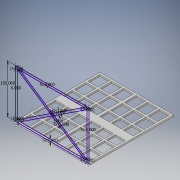
# Autodesk Inventor part: 4 Tape Measures Holder V2
Saved by Autodesk Inventor 2019 (Build 230136000, 136)
## iProperties
Created: 2018-12-28
Part Number: 4 Tape Measures Holder V2
Material: Generic
Document SubType Name: Modeling
Designer: ashle
Density: 1 g/cm^3
Appearance: Default
Author: ashle
Autodesk Inventor part; units mm, degrees
ref_plane "YZ Plane" through (0, 0, 0) normal (1, 0, 0) x (0, 1, 0)
ref_plane "XZ Plane" through (0, 0, 0) normal (0, 1, 0) x (-1, 0, 0)
ref_plane "XY Plane" through (0, 0, 0) normal (0, 0, 1) x (1, 0, 0)
sketch "Sketch1" plane through (0, 0, 0) normal (0, 1, 0) x (-1, 0, 0)
  line L0 (2743.2, 3327.4) -> (-2743.2, 3327.4)
  line L1 (-2743.2, 3327.4) -> (-2743.2, 3175)
  line L2 (-2743.2, 3175) -> (2743.2, 3175)
  line L3 (2743.2, 3175) -> (2743.2, 3327.4)
  line L4 (0, 5131.2687) -> (0, -6149.1862) construction
  line L5 (2743.2, 4620.3571) -> (2743.2, -4424.6448) construction
  line L6 (-2743.2, 4620.3571) -> (-2743.2, -5005.5165) construction
  line L7 (-3643.9458, -3175) -> (3603.587, -3175) construction
  line L8 (3452.6337, 3175) -> (-4564.2023, 3175) construction
  line L9 (-2743.2, 2243.6667) -> (-2743.2, 2091.2667)
  line L10 (2743.2, 2243.6667) -> (-2743.2, 2243.6667)
  line L11 (-2743.2, 2091.2667) -> (2743.2, 2091.2667)
  line L12 (2743.2, 2091.2667) -> (2743.2, 2243.6667)
  line L13 (-2743.2, 1159.9333) -> (-2743.2, 1007.5333)
  line L14 (2743.2, 1159.9333) -> (-2743.2, 1159.9333)
  line L15 (-2743.2, 1007.5333) -> (2743.2, 1007.5333)
  line L16 (2743.2, 1007.5333) -> (2743.2, 1159.9333)
  line L17 (-2743.2, -317.5) -> (2743.2, -317.5)
  line L18 (2743.2, -317.5) -> (2743.2, 317.5)
  line L19 (2743.2, 317.5) -> (-2743.2, 317.5)
  line L20 (-2743.2, 317.5) -> (-2743.2, -317.5)
  line L21 (-2743.2, -317.5) -> (2743.2, 317.5) construction
  line L22 (2743.2, -317.5) -> (-2743.2, 317.5) construction
  line L23 (-101.6, -3327.4) -> (101.6, -3327.4)
  line L24 (101.6, -3327.4) -> (101.6, 3327.4)
  line L25 (101.6, 3327.4) -> (-101.6, 3327.4)
  line L26 (-101.6, 3327.4) -> (-101.6, -3327.4)
  line L27 (-101.6, -3327.4) -> (101.6, 3327.4) construction
  line L28 (101.6, -3327.4) -> (-101.6, 3327.4) construction
  line L29 (3750.9383, 0) -> (-5642.9813, 0) construction
  line L30 (2743.2, -3327.4) -> (-2743.2, -3327.4)
  line L31 (-2743.2, -3327.4) -> (-2743.2, -3175)
  line L32 (-2743.2, -3175) -> (2743.2, -3175)
  line L33 (2743.2, -3175) -> (2743.2, -3327.4)
  line L34 (-2743.2, -2243.6667) -> (-2743.2, -2091.2667)
  line L35 (2743.2, -2243.6667) -> (-2743.2, -2243.6667)
  line L36 (-2743.2, -2091.2667) -> (2743.2, -2091.2667)
  line L37 (2743.2, -2091.2667) -> (2743.2, -2243.6667)
  line L38 (-2743.2, -1159.9333) -> (-2743.2, -1007.5333)
  line L39 (2743.2, -1159.9333) -> (-2743.2, -1159.9333)
  line L40 (-2743.2, -1007.5333) -> (2743.2, -1007.5333)
  line L41 (2743.2, -1007.5333) -> (2743.2, -1159.9333)
  line L42 (2895.6, 3327.4) -> (2743.2, 3327.4)
  line L43 (2743.2, 3327.4) -> (2743.2, -3327.4)
  line L44 (2743.2, -3327.4) -> (2895.6, -3327.4)
  line L45 (2895.6, -3327.4) -> (2895.6, 3327.4)
  line L46 (1803.4, 3327.4) -> (1803.4, -3327.4)
  line L47 (1955.8, -3327.4) -> (1955.8, 3327.4)
  line L48 (1955.8, 3327.4) -> (1803.4, 3327.4)
  line L49 (1803.4, -3327.4) -> (1955.8, -3327.4)
  line L50 (863.6, 3327.4) -> (863.6, -3327.4)
  line L51 (1016, -3327.4) -> (1016, 3327.4)
  line L52 (1016, 3327.4) -> (863.6, 3327.4)
  line L53 (863.6, -3327.4) -> (1016, -3327.4)
  line L54 (-2895.6, 3327.4) -> (-2743.2, 3327.4)
  line L55 (-2743.2, 3327.4) -> (-2743.2, -3327.4)
  line L56 (-2743.2, -3327.4) -> (-2895.6, -3327.4)
  line L57 (-2895.6, -3327.4) -> (-2895.6, 3327.4)
  line L58 (-1803.4, 3327.4) -> (-1803.4, -3327.4)
  line L59 (-1955.8, -3327.4) -> (-1955.8, 3327.4)
  line L60 (-1955.8, 3327.4) -> (-1803.4, 3327.4)
  line L61 (-1803.4, -3327.4) -> (-1955.8, -3327.4)
  line L62 (-863.6, 3327.4) -> (-863.6, -3327.4)
  line L63 (-1016, -3327.4) -> (-1016, 3327.4)
  line L64 (-1016, 3327.4) -> (-863.6, 3327.4)
  line L65 (-863.6, -3327.4) -> (-1016, -3327.4)
  point P0 (0, 0)
  point P1 (-1803.4, 3327.4)
  dimension "d0" = 5486.4
  dimension "d1" = 152.4
  dimension "d5" = 2743.2
  dimension "d6" = 3175
  dimension "d7" = 6350
  dimension "d10" = 1083.7333
  dimension "d15" = 635
  dimension "d16" = 203.2
  dimension "d19" = 2015.0667
  dimension "d20" = 2015.0667
  dimension "d21" = 152.4
  dimension "d24" = 939.8
  dimension "d29" = 1727.2
  dimension "d30" = 1727.2
  dimension "d32" = 939.8
  dimension "d33" = 1083.7333
  dimension "d36" = 152.4
  dimension "d37" = 152.4
  constraints: 132 end point, 28 symmetric about line, 8 collinear, 8 horizontal, 8 parallel, 4 midpoint, 4 perpendicular, 4 vertical, 36 other
  measures "d0" distance of L0.start L0.end
  measures "d1" distance of L2.end L0.start
  measures "d5" distance from line of point (0, 0) L1
  measures "d6" distance from line of point (0, 0) L2
  measures "d7" distance between parallel lines of L7 L8
  measures "d10" distance of L0.end L9.start
  measures "d15" distance between parallel lines of L17 L19
  measures "d16" distance between parallel lines of L26 L24
  measures "d19" distance between parallel lines of L14 L2
  measures "d20" distance between parallel lines of L40 L15
  measures "d21" distance of L42.start L42.end
  measures "d24" distance of L42.end L46.start
  measures "d29" distance between parallel lines of L43 L51
  measures "d30" distance between parallel lines of L62 L50
  measures "d32" distance between parallel lines of L58 L62
  measures "d33" distance between parallel lines of L40 L36
  measures "d36" distance between parallel lines of L35 L36
  measures "d37" distance between parallel lines of L59 L58
extrude "Extrusion1" add sketch "Sketch1" along normal blind 127 contours L3 L2 L47 L0 | L42 L45 L44 L33 L43 L37 L41 L18 L16 L12 L3 | L47 L2 L46 L0 | L46 L2 L51 L0 | L47 L10 L46 L2 | L12 L11 L47 L10 | L51 L2 L50 L0 | L47 L11 L46 L10 | L30 L47 L32 L33 | L50 L2 L24 L0 | L51 L10 L50 L2 | L46 L11 L51 L10 | L47 L14 L46 L11 | L16 L15 L47 L14 | L30 L46 L32 L47 | L24 L2 L26 L0 | L51 L11 L50 L10 | L47 L15 L46 L14 | L30 L51 L32 L46 | L32 L46 L35 L47 | L35 L47 L36 L37 | L26 L2 L62 L0 | L24 L10 L26 L2 | L50 L11 L24 L10 | L51 L14 L50 L11 | L46 L15 L51 L14 | L47 L19 L46 L15 | L18 L17 L47 L19 | L30 L50 L32 L51 | L35 L46 L36 L47 | L62 L2 L63 L0 | L24 L11 L26 L10 | L51 L15 L50 L14 | L47 L17 L46 L19 | L30 L24 L32 L50 | L32 L50 L35 L51 | L35 L51 L36 L46 | L36 L46 L39 L47 | L39 L47 L40 L41 | L63 L2 L58 L0 | L62 L10 L63 L2 | L26 L11 L62 L10 | L24 L14 L26 L11 | L50 L15 L24 L14 | L51 L19 L50 L15 | L46 L17 L51 L19 | L47 L40 L46 L17 | L23 L26 L32 L24 | L35 L50 L36 L51 | L39 L46 L40 L47 | L58 L2 L59 L0 | L62 L11 L63 L10 | L24 L15 L26 L14 | L51 L17 L50 L19 | L30 L62 L32 L26 | L32 L26 L35 L24 | L35 L24 L36 L50 | L36 L50 L39 L51 | L39 L51 L40 L46 | L59 L2 L1 L0 | L58 L10 L59 L2 | L63 L11 L58 L10 | L62 L14 L63 L11 | L26 L15 L62 L14 | L24 L19 L26 L15 | L50 L17 L24 L19 | L51 L40 L50 L17 | L30 L63 L32 L62 | L35 L26 L36 L24 | L39 L50 L40 L51 | L1 L55 L9 L13 L20 L38 L34 L31 L56 L57 L54 | L58 L11 L59 L10 | L62 L15 L63 L14 | L24 L17 L26 L19 | L35 L62 L36 L26 | L32 L63 L35 L62 | L30 L58 L32 L63 | L36 L26 L39 L24 | L39 L24 L40 L50 | L59 L11 L9 L10 | L58 L14 L59 L11 | L63 L15 L58 L14 | L62 L19 L63 L15 | L26 L17 L62 L19 | L24 L40 L26 L17 | L35 L63 L36 L62 | L30 L59 L32 L58 | L39 L26 L40 L24 | L58 L15 L59 L14 | L62 L17 L63 L19 | L39 L62 L40 L26 | L36 L63 L39 L62 | L35 L58 L36 L63 | L32 L59 L35 L58 | L30 L31 L32 L59 | L59 L15 L13 L14 | L58 L19 L59 L15 | L63 L17 L58 L19 | L62 L40 L63 L17 | L39 L63 L40 L62 | L35 L59 L36 L58 | L58 L17 L59 L19 | L39 L58 L40 L63 | L36 L59 L39 L58 | L35 L34 L36 L59 | L59 L17 L20 L19 | L58 L40 L59 L17 | L39 L59 L40 L58 | L39 L38 L40 L59
sketch "Sketch8" plane through (-2895.6, 0, 3327.4) normal (0, 0, 1) x (1, 0, 0)
  line L0 (5791.2, 127) -> (0, 127) construction
  line L1 (0, 127) -> (0, 3937)
  line L2 (0, 3937) -> (5791.2, 3937)
  line L3 (5791.2, 3937) -> (5791.2, 127)
  line L4 (5791.2, 127) -> (0, 3937) construction
  line L5 (0, 127) -> (5791.2, 3937) construction
  line L6 (0, 0) -> (0, 127) construction
  line L7 (5791.2, 0) -> (5791.2, 127) construction
  line L8 (5791.2, 127) -> (0, 127) construction
  line L9 (0, 127) -> (193.04, 127) construction
  line L10 (193.04, 127) -> (193.04, 254) construction
  line L11 (193.04, 254) -> (0, 254) construction
  line L12 (0, 254) -> (0, 127) construction
  line L13 (5791.2, 3937) -> (5598.16, 3937) construction
  line L14 (5598.16, 3937) -> (5598.16, 3810) construction
  line L15 (5598.16, 3810) -> (5791.2, 3810) construction
  line L16 (5791.2, 3810) -> (5791.2, 3937) construction
  line L17 (5791.2, 127) -> (5598.16, 127) construction
  line L18 (5598.16, 127) -> (5598.16, 254) construction
  line L19 (5598.16, 254) -> (5791.2, 254) construction
  line L20 (5791.2, 254) -> (5791.2, 127) construction
  line L21 (0, 3937) -> (193.04, 3937) construction
  line L22 (193.04, 3937) -> (193.04, 3810) construction
  line L23 (193.04, 3810) -> (0, 3810) construction
  line L24 (0, 3810) -> (0, 3937) construction
  line L25 (152.4, 3745.5249) -> (5420.9099, 279.4)
  line L26 (5638.8, 318.4751) -> (370.2901, 3784.6)
  line L27 (5420.9099, 3784.6) -> (152.4, 318.4751)
  line L28 (370.2901, 279.4) -> (5638.8, 3745.5249)
  line L29 (152.4, 3745.5249) -> (152.4, 318.4751)
  line L30 (5638.8, 3745.5249) -> (5638.8, 318.4751)
  line L31 (370.2901, 3784.6) -> (5420.9099, 3784.6)
  line L32 (370.2901, 279.4) -> (5420.9099, 279.4)
  line L33 (5791.2, 0) -> (5791.2, 127) projected
  line L34 (0, 0) -> (0, 127) projected
  line L35 (0, 127) -> (5791.2, 127)
  point P0 (2895.6, 0)
  point P1 (2895.6, 2032)
  point P2 (2895.6, 1940.7881)
  point P3 (3034.2421, 2032)
  point P4 (2895.6, 2123.2119)
  point P5 (2756.9579, 2032)
  dimension "d122" = 3810
  dimension "d125" = 127
  dimension "d126" = 193.04
  dimension "d127" = 127
  dimension "d128" = 193.04
  dimension "d129" = 127
  dimension "d130" = 193.04
  dimension "d131" = 127
  dimension "d132" = 193.04
  dimension "d133" = 152.4
  dimension "d134" = 152.4
  dimension "d135" = 152.4
  dimension "d137" = 76.2
  dimension "d138" = 76.2
  dimension "d139" = 76.2
  dimension "d140" = 76.2
  dimension "d141" = 152.4
  constraints: 62 end point, 14 parallel, 12 coincident, 12 point on line, 6 horizontal, 5 perpendicular, 2 collinear, 2 midpoint
  measures "d122" distance of L0.end L1.end
  measures "d125" distance of L9.end L10.end
  measures "d126" distance of L10.end L11.end
  measures "d127" distance of L13.end L14.end
  measures "d128" distance of L14.end L15.end
  measures "d129" distance of L17.end L18.end
  measures "d130" distance of L18.end L19.end
  measures "d131" distance of L21.end L22.end
  measures "d132" distance of L22.end L23.end
  measures "d133" distance between parallel lines of L1 L29
  measures "d134" distance between parallel lines of L3 L30
  measures "d135" distance between parallel lines of L2 L31
  measures "d137" distance between parallel lines of L4 L25
  measures "d138" distance between parallel lines of L26 L4
  measures "d139" distance between parallel lines of L5 L28
  measures "d140" distance between parallel lines of L27 L5
  measures "d141" distance between parallel lines of L32 L35
equation "\"d0\" = 2 * d5"
equation "\"d7\" = 2 * d6"
equation "\"d10\" = 0.166667 * d7 + 0.166667 * d1"
equation "\"d20\" = d19"
equation "\"d21\" = d1"
equation "\"d24\" = 0.166667 * d0 + 0.166667 * d21"
equation "\"d30\" = d29"
body "Solid1"
